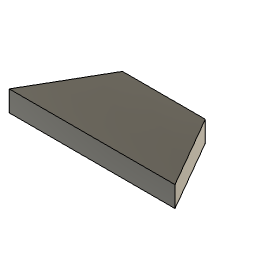
Trapezoid (Autodesk Fusion 360 design; units mm, degrees)
Autodesk Fusion 360 part; units mm, degrees
sketch "Trapezoid" plane through (0, 0, 0) normal (0, 0, 1) x (1, 0, 0)
  line L0 (19.05, 0) -> (6.35, 0)
  line L1 (25.4, -10.9985) -> (19.05, 0)
  line L2 (0, -10.9985) -> (25.4, -10.9985)
  line L3 (6.35, 0) -> (0, -10.9985)
extrude "Extrude1" add sketch "Trapezoid" along normal blind 3.175
